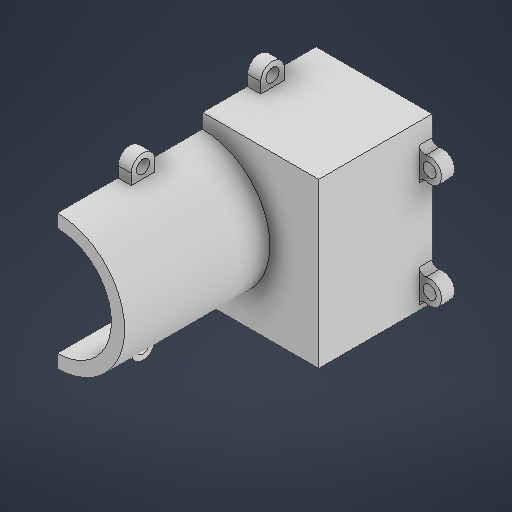
# Autodesk Inventor part: soporte p3
Saved by Autodesk Inventor 2026.1 (Build 301233020, 233B)
## iProperties
Created: 2026-01-16
Part Number: soporte p3
Material: Generic
Document SubType Name: Modeling
Designer: Marcelo
Density: 1 g/cm^3
Appearance: Default
Mass: 58.2542 g
Surface Area: 264.439 cm^2
Volume: 58.2542 cm^3
Author: Marcelo
Autodesk Inventor part; units mm, degrees
ref_plane "YZ Plane" through (0, 0, 0) normal (1, 0, 0) x (0, 1, 0)
ref_plane "XZ Plane" through (0, 0, 0) normal (0, 1, 0) x (-1, 0, 0)
ref_plane "XY Plane" through (0, 0, 0) normal (0, 0, 1) x (1, 0, 0)
sketch "Sketch1" plane through (0, 0, 0) normal (0, 0, 1) x (1, 0, 0)
  line L0 (39, -26) -> (-39, -26)
  line L1 (-39, -26) -> (-39, 26)
  line L2 (-39, 26) -> (39, 26)
  line L3 (39, 26) -> (39, -26)
  line L4 (39, -26) -> (-39, 26) construction
  line L5 (-39, -26) -> (39, 26) construction
  line L6 (44, 31) -> (-44, 31)
  line L7 (-44, 31) -> (-44, -31)
  line L8 (-44, -31) -> (44, -31)
  line L9 (44, -31) -> (44, 31)
  point P0 (0, 0)
  dimension "d0" = 78
  dimension "d1" = 52
  dimension "d2" = 5
  constraints: 20 end point, 4 parallel, 2 midpoint, 2 perpendicular, 1 horizontal, 3 other
  measures "d0" distance of L1.end L2.end
  measures "d1" distance of L0.end L1.end
  measures "d2" distance between parallel lines of L2 L6
extrude "Extrusion1" add sketch "Sketch1" along normal blind 43
sketch "Sketch2" plane through (0, 0, 43) normal (0, 0, 1) x (1, 0, 0)
  line L0 (-44, 31) -> (-44, -31) projected
  line L1 (-44, -31) -> (44, -31) projected
  line L2 (44, -31) -> (44, 31) projected
  line L3 (44, 31) -> (-44, 31) projected
  line L4 (39, -26) -> (-39, -26) projected
  line L5 (-39, -26) -> (-39, 26) projected
  line L6 (-39, 26) -> (39, 26) projected
  line L7 (39, 26) -> (39, -26) projected
  point P0 (0, 0)
extrude "Extrusion2" add sketch "Sketch2" against normal blind 5 contours L3 L2 L1 L0 | L4 L5 L6 L7
sketch "Sketch3" plane through (0, 0, 43) normal (0, 0, 1) x (1, 0, 0)
  circle A0 centre (0, 0) radius 20.5
  dimension "d7" = 41
  constraints: 1 centre point, 1 coincident
  measures "d7" diameter of A0
extrude "Extrusion3" cut sketch "Sketch3" against normal blind 5
sketch "Sketch4" plane through (0, 0, 43) normal (0, 0, 1) x (1, 0, 0)
  circle A0 centre (0, 0) radius 20.5 projected
  circle A1 centre (0, 0) radius 25.5
  dimension "d10" = 5
  constraints: 1 centre point
  measures "d10" radial gap between concentric circles of A0 A1
extrude "Extrusion4" add sketch "Sketch4" along normal blind 55
sketch "Sketch5" plane through (0, 0, 0) normal (1, 0, 0) x (0, 1, 0)
  line L0 (25.5, 43) -> (25.5, 98) projected
  line L1 (31, 0) -> (31, 43) projected
  line L2 (-31, 43) -> (31, 43) projected
  line L3 (-31, 0) -> (31, 0) projected
  line L4 (-31, 0) -> (-31, 43) projected
  line L5 (-25.5, 43) -> (-25.5, 98) projected
  line L6 (25.5, 98) -> (-25.5, 98) projected
  point P0 (0, 0)
extrude "Extrusion5" cut sketch "Sketch5" against normal blind 55
sketch "Sketch7" plane through (0, 0, 0) normal (0, 0, -1) x (-1, 0, 0)
  circle A0 centre (-48, 17) radius 2.5
  circle A1 centre (-48, -23) radius 2.5
  line L0 (-48, 17) -> (-44, 17)
  line L1 (-44, -31) -> (-44, 31) projected
  line L2 (-44, 22.4083) -> (-44, 31)
  line L3 (-48, -23) -> (-44, -23)
  line L4 (-44, 31) -> (0, 31) projected
  line L5 (0, -31) -> (-44, -31) projected
  line L6 (-44, -28.4083) -> (-44, -31)
  line L7 (-44, -17.5917) -> (-44, 10.8153)
  line L8 (-44, 23.1847) -> (-44, 31)
  arc A2 (-46.6154, 21.2817) -> (-46.6154, 12.7183) centre (-48, 17) ccw
  arc A3 (-46.6154, -18.7183) -> (-46.6154, -27.2817) centre (-48, -23) ccw
  line L9 (-44, 19.0616) -> (-44, 31)
  line L10 (-44, -29.1847) -> (-44, -31)
  line L11 (-44, -16.8153) -> (-44, 14.9384)
  arc A4 (-44, 10.8153) -> (-46.6154, 12.7183) centre (-46, 10.8153) ccw
  arc A5 (-46.6154, 21.2817) -> (-44, 23.1847) centre (-46, 23.1847) ccw
  arc A6 (-44, -29.1847) -> (-46.6154, -27.2817) centre (-46, -29.1847) ccw
  arc A7 (-46.6154, -18.7183) -> (-44, -16.8153) centre (-46, -16.8153) ccw
  point P0 (0, 0)
  point P1 (-44, 15.1972)
  point P2 (-44, -24.8028)
  point P3 (-44, -21.1972)
  point P4 (-44, -25.0616)
  point P5 (-44, -20.9384)
  dimension "d40" = 5
  dimension "d45" = 4
  dimension "d46" = 5
  dimension "d68" = 40
  dimension "d75" = 8
  dimension "d76" = 4
  dimension "d77" = 2
  dimension "d78" = 2
  dimension "d79" = 2
  constraints: 18 end point, 16 point on circle, 8 centre point, 8 tangent, 5 point on line, 4 collinear, 3 equal radius, 2 horizontal, 2 vertical, 1 perpendicular, 10 other
  measures "d40" diameter of A1
  measures "d45" distance of L3.start L3.end
  measures "d46" diameter of A0
  measures "d68" distance between parallel lines of L0 L3
  measures "d75" distance between parallel lines of L5 L3
  measures "d76" distance of L0.start L0.end
  measures "d77" radial gap between concentric circles of A2 A0
  measures "d78" radial gap between concentric circles of A1 A3
  measures "d79" radius of A4
extrude "Extrusion7" add sketch "Sketch7" against normal blind 5
sketch "Sketch10" plane through (0, 0, 0) normal (-1, 0, 0) x (0, 0, 1)
  circle A0 centre (21.5, 35) radius 2.5
  line L0 (0, 26) -> (0, 31) projected
  line L1 (0, 31) -> (43, 31) projected
  arc A1 (26, 35) -> (17, 35) centre (21.5, 35) ccw
  line L2 (43, 25.5) -> (98, 25.5) projected
  circle A2 centre (70.5, 29.5) radius 2.5
  arc A3 (75, 29.5) -> (66, 29.5) centre (70.5, 29.5) ccw
  line L3 (0, -31) -> (43, -31) projected
  line L4 (21.5, -31) -> (21.5, -35)
  circle A4 centre (21.5, -35) radius 2.5
  arc A5 (17, -35) -> (26, -35) centre (21.5, -35) ccw
  line L5 (43, -25.5) -> (98, -25.5) projected
  line L6 (70.5, -25.5) -> (70.5, -29.5)
  circle A6 centre (70.5, -29.5) radius 2.5
  arc A7 (66, -29.5) -> (75, -29.5) centre (70.5, -29.5) ccw
  line L7 (0, -31) -> (16.0917, -31)
  line L8 (26.9083, -31) -> (43, -31)
  line L9 (43, -25.5) -> (65.0917, -25.5)
  line L10 (43, -31) -> (43, 31) projected
  line L11 (75.9083, -25.5) -> (98, -25.5)
  line L12 (0, 31) -> (16.0917, 31)
  line L13 (26.9083, 31) -> (43, 31)
  line L14 (65.0917, 25.5) -> (43, 25.5)
  line L15 (75, 25.5) -> (98, 25.5)
  line L16 (98, 20.5) -> (98, -20.5) projected
  line L17 (70.5, 29.5) -> (70.5, 25.5)
  line L18 (98, 25.5) -> (98, 20.5) projected
  line L19 (21.5, 35) -> (21.5, 31)
  line L20 (16.0917, 31) -> (0, 31)
  line L21 (65.0917, 25.5) -> (43, 25.5)
  line L22 (75, 25.5) -> (98, 25.5)
  line L23 (75.9083, -25.5) -> (98, -25.5)
  line L24 (65.0917, -25.5) -> (43, -25.5)
  line L25 (26.9083, -31) -> (43, -31)
  line L26 (16.0917, -31) -> (0, -31)
  line L27 (17, 35) -> (17, 31)
  line L28 (26, 35) -> (26, 31)
  line L29 (66, 25.5) -> (66, 29.5)
  line L30 (75, 25.5) -> (75, 29.5)
  line L31 (26, -35) -> (26, -31)
  line L32 (17, -35) -> (17, -31)
  line L33 (75, -29.5) -> (75, -25.5)
  line L34 (66, -29.5) -> (66, -25.5)
  point P0 (0, 0)
  point P1 (19.4384, 31)
  point P2 (23.5616, 31)
  point P3 (68.4384, 25.5)
  point P4 (72.5616, 25.5)
  point P5 (23.5616, -31)
  point P6 (19.4384, -31)
  point P7 (72.5616, -25.5)
  point P8 (68.4384, -25.5)
  point P9 (26, -31)
  point P10 (17, -31)
  dimension "d52" = 5
  dimension "d56" = 2
  dimension "d57" = 5
  dimension "d58" = 2
  dimension "d59" = 4
  dimension "d60" = 5
  dimension "d61" = 2
  dimension "d70" = 27.5
  dimension "d71" = 4
  dimension "d72" = 27.5
  dimension "d73" = 4
  dimension "d74" = 90
  dimension "d80" = 4
  dimension "d81" = 2
  dimension "d82" = 5
  constraints: 54 end point, 23 point on line, 16 point on circle, 10 perpendicular, 8 centre point, 8 tangent, 6 collinear, 4 coincident, 4 midpoint, 4 vertical, 3 parallel
  measures "d52" diameter of A0
  measures "d56" radial gap between concentric circles of A0 A1
  measures "d57" diameter of A2
  measures "d58" radial gap between concentric circles of A2 A3
  measures "d59" distance of L4.start L4.end
  measures "d60" diameter of A4
  measures "d61" radial gap between concentric circles of A4 A5
  measures "d70" distance between parallel lines of L16 L6
  measures "d71" distance of L17.start L17.end
  measures "d72" distance between parallel lines of L18 L17
  measures "d73" distance of L19.start L19.end
  measures "d74" angle of L1 L19
  measures "d80" distance of L6.start L6.end
  measures "d81" radial gap between concentric circles of A7 A6
  measures "d82" diameter of A6
extrude "Extrusion8" add sketch "Sketch10" against normal blind 5
body "Solid1"
